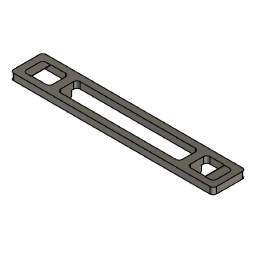
125mm 2020 Bed Frame Spacer v4 (Autodesk Fusion 360 design; units mm, degrees)
Autodesk Fusion 360 part; units mm, degrees
sketch "Sketch1" plane through (0, 0, 0) normal (0, 0, 1) x (1, 0, 0)
  line L0 (2, 0) -> (123, 0)
  line L1 (125, 2) -> (125, 18)
  line L2 (123, 20) -> (2, 20)
  line L3 (0, 18) -> (0, 2)
  arc A0 (2, 20) -> (0, 18) centre (2, 18) ccw
  arc A1 (0, 2) -> (2, 0) centre (2, 2) ccw
  arc A2 (123, 0) -> (125, 2) centre (123, 2) ccw
  arc A3 (125, 18) -> (123, 20) centre (123, 18) ccw
  line L4 (4, 4) -> (121, 4)
  line L5 (121, 4) -> (121, 16)
  line L6 (121, 16) -> (4, 16)
  line L7 (4, 16) -> (4, 4)
  line L8 (20, 16) -> (25, 16)
  line L9 (25, 16) -> (25, 4)
  line L10 (25, 4) -> (20, 4)
  line L11 (20, 4) -> (20, 16)
  line L12 (62.5, 0) -> (62.5, 20) construction
  line L13 (105, 4) -> (105, 16)
  line L14 (105, 16) -> (100, 16)
  line L15 (100, 4) -> (105, 4)
  line L16 (100, 16) -> (100, 4)
  line L17 (20, 12.75) -> (105, 12.75)
  line L18 (105, 12.75) -> (105, 7.25)
  line L19 (105, 7.25) -> (20, 7.25)
  line L20 (20, 7.25) -> (20, 12.75)
  line L21 (20, 12.75) -> (105, 7.25) construction
  line L22 (105, 12.75) -> (20, 7.25) construction
  line L23 (9, 16) -> (9, 4)
  line L24 (116, 16) -> (116, 4)
  point P0 (125, 0)
  point P1 (0, 20)
  point P2 (62.5, 10)
  dimension "d1" = 125
  dimension "d2" = 20
  dimension "d3" = 2
  dimension "d4" = -4
  dimension "d5" = 5
  dimension "d7" = 80
  dimension "d16" = 5.5
  dimension "d23" = 5
  dimension "d24" = 5
  constraint horizontal L0
  constraint vertical L1
  constraint horizontal L2
  constraint vertical L3
  constraint coincident P1 L2
  constraint coincident P1 L3
  constraint tangent L2 A0
  constraint tangent L3 A0
  constraint coincident origin L0
  constraint coincident origin L3
  constraint tangent L0 A1
  constraint tangent L3 A1
  constraint equal A0 A1
  constraint coincident P0 L0
  constraint coincident P0 L1
  constraint tangent L0 A2
  constraint tangent L1 A2
  constraint equal A0 A2
  constraint tangent L1 A3
  constraint tangent L2 A3
  constraint equal A0 A3
  constraint horizontal L8
  constraint vertical L9
  constraint horizontal L10
  constraint vertical L11
  constraint coincident L4 L9.end
  constraint coincident L6 L8.start
  constraint midpoint L0 L12.start
  constraint perpendicular L2 L12
  constraint symmetric L8.start L12 L13.end
  constraint symmetric L8.end L12 L14.end
  constraint symmetric L9.end L12 L15.start
  constraint symmetric L10.end L12 L13.start
  constraint midpoint L2 L12.end
  constraint horizontal L17
  constraint perpendicular L17 L18
  constraint parallel L17 L19
  constraint parallel L18 L20
  constraint coincident L11 L17.start
  constraint coincident L21 P2
  constraint coincident L22 P2
  constraint midpoint L12 P2
  constraint coincident L6 L23.start
  constraint coincident L4 L23.end
  constraint perpendicular L4 L23
  constraint coincident L6 L24.start
  constraint coincident L4 L24.end
  constraint perpendicular L4 L24
  measures "d1" distance of origin P0
  measures "d2" distance of origin P1
  measures "d3" radius of A0
  measures "d5" distance of L9 L11
  measures "d7" distance of L9 L13
  measures "d16" distance of L17 L19
  measures "d23" distance of L7 L23
  measures "d24" distance of L5 L24
extrude "Extrude1" add sketch "Sketch1" along normal blind 4 contours L0 L1 L2 L3 A0 A1 A2 A3 | L4 L9 L10 L11 L19 | L9 L11 L17 L19 L20 | L6 L8 L9 L11 L17 | L4 L13 L15 L16 L19 | L13 L16 L17 L18 L19 | L6 L13 L14 L16 L17
extrude "Extrude3" add sketch "Sketch1" against normal blind 4 contours L9 L11 L17 L19 L20 | L13 L16 L17 L18 L19
extrude "Extrude4" add sketch "Sketch1" against normal blind 0.2 from surface at 4 contours L4 L6 L7 L23 | L4 L5 L6 L24
fillet "Fillet1" radius 1 4 edges at (22.5, 12.75, -4) (22.5, 7.25, -4) (102.5, 12.75, -4) (102.5, 7.25, -4)
fillet "Fillet2" radius 2 12 edges at (121, 4, 2) (105, 4, 2) (100, 4, 2) (121, 16, 2) (105, 16, 2) (100, 16, 2) (20, 4, 2) (4, 4, 2) (4, 16, 2) (20, 16, 2) (25, 4, 2) (25, 16, 2)
